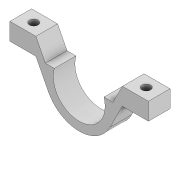
# Autodesk Inventor part: Motor_mount_clamp_p1
Saved by Autodesk Inventor 2022 (Build 260153000, 153)
## iProperties
Created: 2022-04-28
Part Number: Motor_mount_clamp_p1
Material: Generic
Document SubType Name: Modeling
Designer: dell
Density: 1 g/cm^3
Appearance: Default
Author: dell
Autodesk Inventor part; units mm, degrees
ref_plane "YZ Plane" through (0, 0, 0) normal (1, 0, 0) x (0, 1, 0)
ref_plane "XZ Plane" through (0, 0, 0) normal (0, 1, 0) x (-1, 0, 0)
ref_plane "XY Plane" through (0, 0, 0) normal (0, 0, 1) x (1, 0, 0)
sketch "Sketch1" plane through (0, 0, 0) normal (0, 0, 1) x (1, 0, 0)
  circle A0 centre (0, 0) radius 6
  circle A1 centre (0, 0) radius 8
  line L0 (-16, 8) -> (16, 8)
  line L1 (16, 8) -> (16, 6)
  line L2 (16, 6) -> (-16, 6)
  line L3 (-16, 6) -> (-16, 8)
  line L4 (-16, 6) -> (-10, 6)
  line L5 (-10, 6) -> (-10, 2)
  line L6 (-10, 2) -> (-16, 2)
  line L7 (-16, 2) -> (-16, 6)
  line L8 (16, 6) -> (10, 6)
  line L9 (10, 6) -> (10, 2)
  line L10 (10, 2) -> (16, 2)
  line L11 (16, 2) -> (16, 6)
  line L12 (-10, 2) -> (-7.1269, -3.6343)
  line L13 (-10, 6) -> (-7.8143, 1.7138)
  line L14 (10, 6) -> (7.8143, 1.7138)
  line L15 (10, 2) -> (7.1269, -3.6343)
  arc A2 (-6.6518, 4.4444) -> (-7.4833, 6) centre (-7.4833, 5) ccw
  arc A3 (7.4833, 6) -> (6.6518, 4.4444) centre (7.4833, 5) ccw
  line L16 (-7.8143, 1.7138) -> (-5.75, 1.7138)
  line L17 (7.8143, 1.7138) -> (5.75, 1.7138)
  line L18 (-13, -5.2365) -> (-13, 13.2519) construction
  line L19 (13, -7.3842) -> (13, 14.4806) construction
  point P0 (-10, 6)
  point P1 (10, 6)
  dimension "d12" = 12
  dimension "d13" = 2
  dimension "d14" = 16
  dimension "d15" = 16
  dimension "d16" = 6
  dimension "d17" = 4
  dimension "d18" = 6
  dimension "d19" = 4
  dimension "d20" = 1
  dimension "d21" = 1
  dimension "d39" = 13
  dimension "d40" = 13
  constraints: 40 end point, 12 point on circle, 8 parallel, 8 tangent, 4 centre point, 4 horizontal, 3 perpendicular, 3 point on line, 2 vertical, 1 coincident
  measures "d12" diameter of A0
  measures "d13" radial gap between concentric circles of A0 A1
  measures "d14" distance from line of L3 A0.centre
  measures "d15" distance from line of A0.centre L1
  measures "d16" distance of L9.end L10.end
  measures "d17" distance of L8.end L9.end
  measures "d18" distance of L5.end L6.end
  measures "d19" distance of L4.end L5.end
  measures "d20" radius of A2
  measures "d21" radius of A3
  measures "d39" distance from line of A0.centre L19
  measures "d40" distance from line of A0.centre L18
extrude "Extrusion1" add sketch "Sketch1" against normal blind 5 contours A0 L17 A1 L16 | L14 L9 L15 A1 | A1 L12 L5 L13 | L2 L11 L10 L9 | L5 L6 L7 L2
sketch "Sketch4" plane through (-16, 6, 0) normal (0, 1, 0) x (1, 0, 0)
  circle A0 centre (3, 2.5) radius 1
  circle A1 centre (29, 2.5) radius 1
  line L0 (0, 0) -> (0, 5) projected
  line L1 (32, 0) -> (32, 5) projected
  line L2 (32, 0) -> (26, 0) projected
  line L3 (6, 0) -> (0, 0) projected
  point P0 (16, 0)
  dimension "d41" = 2
  dimension "d42" = 2
  dimension "d43" = 3
  dimension "d44" = 3
  dimension "d45" = 2.5
  dimension "d46" = 2.5
  constraints: 2 centre point
  measures "d41" diameter of A0
  measures "d42" diameter of A1
  measures "d43" distance from line of L0 A0.centre
  measures "d44" distance from line of L1 A1.centre
  measures "d45" distance from line of L2 A1.centre
  measures "d46" distance from line of L3 A0.centre
extrude "Extrusion4" cut sketch "Sketch4" against normal blind 5
equation "\"d15\" = d14"
body "Solid1"
